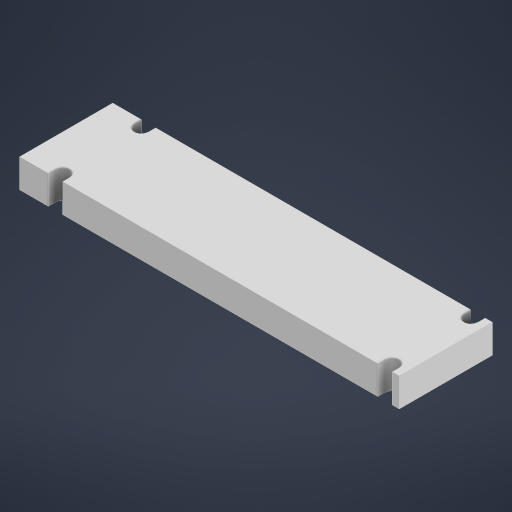
# Autodesk Inventor part: Langbektang houder
Saved by Autodesk Inventor 2023.2 (Build 272271000, 271)
## iProperties
Created: 2020-09-09
Part Number: Langbektang houder
Material: Generic
Document SubType Name: Modeling
Designer: nathan.bollaert
Density: 1 g/cm^3
Appearance: Default
Author: nathan.bollaert
Autodesk Inventor part; units mm, degrees
ref_plane "YZ Plane" through (0, 0, 0) normal (1, 0, 0) x (0, 1, 0)
ref_plane "XZ Plane" through (0, 0, 0) normal (0, 1, 0) x (-1, 0, 0)
ref_plane "XY Plane" through (0, 0, 0) normal (0, 0, 1) x (1, 0, 0)
sketch "Sketch1" plane through (0, 0, 0) normal (0, 1, 0) x (-1, 0, 0)
  line L0 (0, 0) -> (53, 0)
  line L1 (53, 0) -> (53, -13)
  line L2 (53, -13) -> (0, -13)
  line L3 (0, -13) -> (0, 0)
  circle A0 centre (48, -12) radius 1
  circle A1 centre (48, -1) radius 1
  line L4 (53, -6.5) -> (0, -6.5)
  line L5 (26.5, 0) -> (26.5, -13)
  circle A2 centre (2, -12) radius 1
  circle A3 centre (2, -1) radius 1
  line L6 (49, -1) -> (49, 0)
  line L7 (47, -1) -> (47, 0)
  circle A4 centre (48, -12) radius 1
  line L8 (49, -12) -> (49, -13)
  line L9 (47, -12) -> (47, -13)
  line L10 (1, -1) -> (1, 0)
  line L11 (3, -1) -> (3, 0)
  circle A5 centre (2, -12) radius 1
  line L12 (1, -12) -> (1, -13)
  line L13 (3, -12) -> (3, -13)
  point P0 (3, -12)
  dimension "d228" = 13
  dimension "d229" = 53
  dimension "d233" = 5
  dimension "d234" = 2
  dimension "d235" = 11
  dimension "d237" = 2
  constraints: 28 end point, 10 symmetric about line, 8 point on circle, 6 centre point, 4 midpoint, 4 perpendicular, 4 point on line, 4 tangent, 2 parallel, 2 vertical alignment, 1 equal radius, 1 horizontal, 1 horizontal alignment, 1 vertical, 4 other
  measures "d228" distance of L0.end L1.end
  measures "d229" distance of L1.end L2.end
  measures "d233" distance from line of L1 A0.centre
  measures "d234" diameter of A0
  measures "d235" distance of A2.centre A3.centre
  measures "d237" distance from line of L3 A3.centre
extrude "Extrusion1" add sketch "Sketch1" against normal blind 4 contours L0 L10 A3 L11 L5 L4 L3 | L4 L5 L2 L13 A2 L12 L3 | L5 L0 L7 A1 L6 L1 L4 | L4 L1 L2 L8 A0 L9 L5
body "Solid5"
